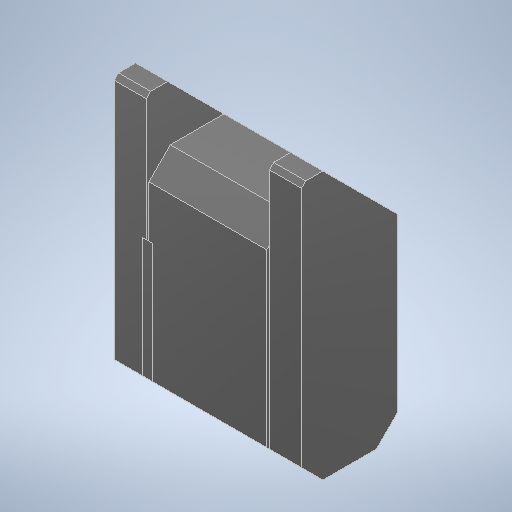
# Autodesk Inventor part: 3D_jigu
Saved by Autodesk Inventor 2025 (Build 290162000, 162)
## iProperties
Created: 2024-07-24
Part Number: 3D_jigu
Material: 一般
Document SubType Name: Modeling
Designer: 8326d
Density: 1 g/cm^3
Appearance: 滑らか - 黒
Author: 8326d
## iProperties of the stored document 3D_jigu_3D プリント.ipt
Created: 2024-07-24
Part Number: 3D_jigu_3D プリント
Material: 一般
Document SubType Name: Modeling
Designer: 8326d
Density: 1 g/cm^3
Appearance: 既定
Author: 8326d
Autodesk Inventor part; units mm, degrees
ref_plane "YZ Plane" through (0, 0, 0) normal (1, 0, 0) x (0, 1, 0)
ref_plane "XZ Plane" through (0, 0, 0) normal (0, 1, 0) x (-1, 0, 0)
ref_plane "XY Plane" through (0, 0, 0) normal (0, 0, 1) x (1, 0, 0)
sketch "スケッチ1" plane through (0, 0, 0) normal (0, 0, 1) x (1, 0, 0)
  line L0 (-5.5, -10) -> (5.5, -10)
  line L1 (5.5, -10) -> (5.5, 10)
  line L2 (5.5, 10) -> (-5.5, 10)
  line L3 (-5.5, 10) -> (-5.5, -10)
  line L4 (-5.5, -10) -> (5.5, 10) construction
  line L5 (5.5, -10) -> (-5.5, 10) construction
  point P0 (0, 0)
  dimension "d0" = 11
  dimension "d1" = 20
  constraints: 12 end point, 2 midpoint, 2 parallel, 1 horizontal, 1 perpendicular
  measures "d0" distance of L2.end L1.end
  measures "d1" distance of L1.end L0.end
extrude "押し出し1" add sketch "スケッチ1" along normal mid plane 9
sketch "スケッチ2" plane through (5.5, -10, 4.5) normal (1, 0, 0) x (0, 0, -1)
  circle A0 centre (4.5, 5) radius 2.75
  point P0 (4.5, 10)
  dimension "d4" = 5.5
  dimension "d5" = 5
  constraints: 1 centre point, 1 vertical alignment
  measures "d4" diameter of A0
  measures "d5" distance of point (4.5, 10) A0.centre
extrude "押し出し2" cut sketch "スケッチ2" against normal through all
sketch "スケッチ3" plane through (-5.5, -10, 4.5) normal (-1, 0, 0) x (0, 0, 1)
  point P0 (-4.5, 10)
  point P1 (-4.5, 15)
  dimension "d8" = 5
  constraints: 1 vertical alignment
  measures "d8" distance of point (-4.5, 15) point (-4.5, 10)
hole "穴1" at (-5.5, 5, 0) direction (1, 0, 0) diameter 4 end through all
sketch "スケッチ4" plane through (0, 0, 0) normal (1, 0, 0) x (0, 1, 0)
  circle A0 centre (5, 0) radius 2 projected
  circle A1 centre (5, 0) radius 1.7
  point P0 (0, 0)
  dimension "d16" = 0.3
  constraints: 1 centre point
  measures "d16" radial gap between concentric circles of A0 A1
extrude "押し出し3" add sketch "スケッチ4" along normal mid plane 11.5 contours A1
sketch "スケッチ5" plane through (-5.75, 5, 0) normal (-1, 0, 0) x (0, 0, 1)
  line L0 (4.5, 5) -> (4.5, -15) projected
  line L1 (-4.5, 5) -> (4.5, 5) projected
  line L2 (-4.5, -15) -> (-4.5, 5) projected
  line L3 (-4.5, -15) -> (4.5, -15) projected
  circle A0 centre (0, -10) radius 2.75 projected
  point P0 (0, -5)
extrude "押し出し4" add sketch "スケッチ5" along normal blind 3
sketch "スケッチ6" plane through (5.75, 5, 0) normal (1, 0, 0) x (0, 0, -1)
  line L0 (4.5, 5) -> (4.5, -15) projected
  line L1 (4.5, 5) -> (-4.5, 5) projected
  line L2 (-4.5, -15) -> (-4.5, 5) projected
  line L3 (-4.5, -15) -> (4.5, -15) projected
  point P0 (0, -5)
extrude "押し出し5" add sketch "スケッチ6" along normal blind 3
chamfer "面取り1" distance 1 angle 45 2 edges at (-5.5, 5, -2) (5.5, 5, -2)
chamfer "面取り2" distance 1.2 angle 45 2 edges at (5.75, 3.3, 0) (-5.75, 3.3, 0)
sketch "スケッチ7" plane through (-5.75, -10, -4.5) normal (0, 0, -1) x (-1, 0, 0)
  line L0 (-0.25, 7.75) -> (-0.25, 2.25) projected
  line L1 (0, 7.75) -> (0, 2.25) projected
  line L2 (-0.25, 5) -> (0, 5) construction
  line L3 (-0.625, -2) -> (0.375, -2)
  line L4 (0.375, -2) -> (0.375, 12)
  line L5 (0.375, 12) -> (-0.625, 12)
  line L6 (-0.625, 12) -> (-0.625, -2)
  line L7 (-0.625, -2) -> (0.375, 12) construction
  line L8 (0.375, -2) -> (-0.625, 12) construction
  point P0 (-5.75, 10)
  point P1 (-0.125, 5)
  dimension "d29" = 1
  dimension "d30" = 14
  constraints: 14 end point, 5 midpoint, 2 parallel, 1 horizontal, 1 perpendicular
  measures "d29" distance of L5.end L4.end
  measures "d30" distance of L4.end L3.end
extrude "押し出し6" cut sketch "スケッチ7" against normal through all
chamfer "面取り3" distance 1.2 angle 45 4 edges at (-5.3125, 2, 4.5) (-5.9375, 2, 4.5) (-5.9375, 2, -4.5) (-5.3125, 2, -4.5)
chamfer "面取り4" distance 2 angle 45 10 edges at (-7.4375, -10, 4.5) (0.1875, -10, 4.5) (7.25, -10, 4.5) (7.25, -10, -4.5) (0.1875, -10, -4.5) (-7.4375, -10, -4.5) (7.25, 10, -4.5) (0, 10, -4.5) (-7.25, 10, -4.5) (0, 10, 4.5)
sketch "スケッチ8" plane through (-8.75, 5, 0) normal (-1, 0, 0) x (0, 0, 1)
  line L0 (4.5, 5) -> (-2.5, 5) projected
  line L1 (4.5, -13) -> (4.5, 5) projected
  line L2 (-2.5, 5) -> (-4.5, 3) projected
  line L3 (-2.5, 5) -> (2.5, 10)
  line L4 (2.5, 10) -> (4.5, 10)
  line L5 (4.5, 10) -> (4.5, 5)
  point P0 (0, -5)
  dimension "d39" = 5
  constraints: 6 end point, 1 collinear, 1 horizontal, 1 perpendicular
  measures "d39" distance between parallel lines of L0 L4
extrude "押し出し7" add sketch "スケッチ8" against normal up to surface (3 mm away)
chamfer "面取り5" distance 0.4 angle 45 1 edges at (-7.25, 15, 4.5)
mirror "ミラー1" about plane through (0, 0, 0) normal (1, 0, 0) of "押し出し7", "面取り5"
